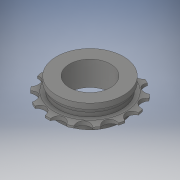
# Autodesk Inventor part: roue libre
Saved by Autodesk Inventor 2018.1 (Build 221171000, 171)
## iProperties
Created: 2022-05-13
Part Number: roue libre
Material: Generic
Document SubType Name: Modeling
Designer: Bureau
Density: 1 g/cm^3
Appearance: Default
Author: Bureau
Autodesk Inventor part; units mm, degrees
ref_plane "YZ Plane" through (0, 0, 0) normal (1, 0, 0) x (0, 1, 0)
ref_plane "XZ Plane" through (0, 0, 0) normal (0, 1, 0) x (-1, 0, 0)
ref_plane "XY Plane" through (0, 0, 0) normal (0, 0, 1) x (1, 0, 0)
sketch "Sketch1" plane through (0, 0, 0) normal (1, 0, 0) x (0, 1, 0)
  line L0 (0, 0) -> (0, -10)
  line L1 (0, 0) -> (15, 0)
  line L2 (15, 0) -> (15, -18)
  line L3 (15, -18) -> (23, -18)
  line L4 (23, -18) -> (23, -13)
  line L5 (23, -13) -> (26, -13)
  line L6 (30.9522, -12.1268) -> (30.9522, -10.6732)
  line L7 (26, -9.8) -> (23, -9.8)
  line L8 (15, 0) -> (24.5, 0)
  line L9 (24.5, 0) -> (24.5, -4)
  line L10 (23, -9.8) -> (23, -6.8)
  line L11 (23, -6.8) -> (24.5, -4)
  line L12 (23, -9.8) -> (26, -9.8)
  line L13 (26, -9.8) -> (30.9522, -10.6732)
  line L14 (26, -13) -> (30.9522, -12.1268)
  line L15 (26, -13) -> (31.0286, -13) construction
  point P0 (23, -2.8)
  point P1 (24.6166, 0)
  dimension "d0" = 10
  dimension "d1" = 15
  dimension "d2" = 18
  dimension "d3" = 8
  dimension "d4" = 5
  dimension "d7" = 7
  dimension "d10" = 23
  dimension "d11" = 9.5
  dimension "d12" = 4
  dimension "d13" = 3
  dimension "d14" = 3
  dimension "d15" = 170
  dimension "d16" = 10
  constraints: 32 end point, 7 perpendicular, 3 horizontal, 3 point on line, 2 vertical, 1 equal length
  measures "d0" distance of L0.start L0.end
  measures "d1" distance of L0.start L1.end
  measures "d2" distance of L1.end L2.end
  measures "d3" distance of L2.end L3.end
  measures "d4" distance of L3.end L4.end
  measures "d7" distance of L7.end point (23, -2.8)
  measures "d10" distance from line of L0 L3.end
  measures "d11" distance of L1.end L8.end
  measures "d12" distance of L8.end L9.end
  measures "d13" distance of L7.end L10.end
  measures "d14" distance of L7.start L7.end
  measures "d15" angle of L12 L13
  measures "d16" angle of L15 L14
revolve "Revolution1" add sketch "Sketch1" angle 360 about axis through (0, 0, 0) along (0, 0, -1)
sketch "Sketch2" plane through (0, 0, -13) normal (0, 0, -1) x (-1, 0, 0)
  circle A0 centre (0, 0) radius 30.9522 projected
  line L0 (-30.9522, 0) -> (-30.9522, 5)
  line L1 (-30.9522, 5) -> (-30.9522, -5)
  arc A1 (-30.9522, -5) -> (-30.9522, 5) centre (-31.6312, 0) ccw
  arc A2 (-25.7176, -17.9345) -> (-30.0564, -8.9248) centre (-28.4987, -13.7242) ccw
  arc A3 (-15.3892, -27.3169) -> (-23.2075, -21.082) centre (-19.7217, -24.7302) ccw
  arc A4 (-2.0129, -31.2888) -> (-11.7622, -29.0636) centre (-7.0386, -30.8381) ccw
  arc A5 (11.7622, -29.0636) -> (2.0129, -31.2888) centre (7.0386, -30.8381) ccw
  arc A6 (23.2075, -21.082) -> (15.3892, -27.3169) centre (19.7217, -24.7302) ccw
  arc A7 (30.0564, -8.9248) -> (25.7176, -17.9345) centre (28.4987, -13.7242) ccw
  arc A8 (30.9522, 5) -> (30.9522, -5) centre (31.6312, 0) ccw
  arc A9 (25.7176, 17.9345) -> (30.0564, 8.9248) centre (28.4987, 13.7242) ccw
  arc A10 (15.3892, 27.3169) -> (23.2075, 21.082) centre (19.7217, 24.7302) ccw
  arc A11 (2.0129, 31.2888) -> (11.7622, 29.0636) centre (7.0386, 30.8381) ccw
  arc A12 (-11.7622, 29.0636) -> (-2.0129, 31.2888) centre (-7.0386, 30.8381) ccw
  arc A13 (-23.2075, 21.082) -> (-15.3892, 27.3169) centre (-19.7217, 24.7302) ccw
  arc A14 (-30.0564, 8.9248) -> (-25.7176, 17.9345) centre (-28.4987, 13.7242) ccw
  arc A15 (-25.3918, -17.7002) -> (-22.9066, -20.8165) centre (0, 0) ccw
  arc A16 (-15.1974, -26.9644) -> (-11.6062, -28.6938) centre (0, 0) ccw
  arc A17 (-30.557, -4.9302) -> (-29.6701, -8.8162) centre (0, 0) ccw
  arc A18 (-29.6701, 8.8162) -> (-30.557, 4.9302) centre (0, 0) ccw
  arc A19 (-22.9066, 20.8165) -> (-25.3918, 17.7002) centre (0, 0) ccw
  arc A20 (-11.6062, 28.6938) -> (-15.1974, 26.9644) centre (0, 0) ccw
  arc A21 (1.993, 30.888) -> (-1.993, 30.888) centre (0, 0) ccw
  arc A22 (15.1974, 26.9644) -> (11.6062, 28.6938) centre (0, 0) ccw
  arc A23 (25.3918, 17.7002) -> (22.9066, 20.8165) centre (0, 0) ccw
  arc A24 (30.557, 4.9302) -> (29.6701, 8.8162) centre (0, 0) ccw
  arc A25 (29.6701, -8.8162) -> (30.557, -4.9302) centre (0, 0) ccw
  arc A26 (22.9066, -20.8165) -> (25.3918, -17.7002) centre (0, 0) ccw
  arc A27 (-1.993, -30.888) -> (1.993, -30.888) centre (0, 0) ccw
  arc A28 (11.6062, -28.6938) -> (15.1974, -26.9644) centre (0, 0) ccw
  dimension "d17" = 5
  dimension "d18" = 10
  dimension "d22" = 360
  constraints: 84 point on circle, 28 centre point, 4 end point, 3 coincident, 2 vertical, 1 horizontal alignment, 1 point on line, 70 other
  measures "d17" distance of L0.start L0.end
  measures "d18" distance of L0.end L1.end
extrude "Extrusion1" cut sketch "Sketch2" against normal blind 10 contours A0 A8 | A9 A0 | A0 A7 | A10 A0 | A0 A6 | A11 A0 | A0 A5 | A12 A0 | A0 A4 | A13 A0 | A0 A3 | A14 A0 | A0 A2 | A1 A0
body "Solid1"
